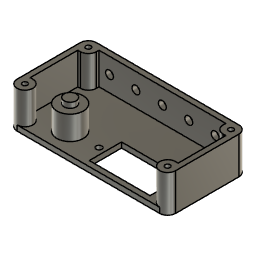
TRGRIP01_Base_Top_60x30x14 (Autodesk Fusion 360 design; units mm, degrees)
Autodesk Fusion 360 part; units mm, degrees
sketch "스케치1" plane through (0, 0, 0) normal (0, 0, 1) x (1, 0, 0)
  line L0 (0, 0) -> (60, 0)
  line L1 (60, 0) -> (60, 30)
  line L2 (60, 30) -> (0, 30)
  line L3 (0, 30) -> (0, 0)
  dimension "d1" = 60
  dimension "d2" = 30
  constraint horizontal L0
  constraint vertical L1
  constraint horizontal L2
  constraint vertical L3
  constraint coincident L0.start L3.end
  measures "d1" distance of L0.start L0.end
  measures "d2" distance of L0.start L2.end
extrude "돌출1" add sketch "스케치1" along normal blind 2
sketch "스케치2" plane through (0, 0, 2) normal (0, 0, 1) x (-1, 0, 0)
  circle A0 centre (-53.75, -8.1) radius 1.1
  circle A1 centre (-25.95, -8.1) radius 1.1
  circle A2 centre (-15, -8.1) radius 5
  line L0 (0, 0) -> (-60, 0)
  line L1 (-51.35, -2) -> (-51.35, -14.2)
  line L2 (-51.35, -14.2) -> (-28.35, -14.2)
  line L3 (-28.35, -14.2) -> (-28.35, -2)
  line L4 (-51.35, -2) -> (-28.35, -2)
  dimension "d5" = 2.2
  dimension "d6" = 27.8
  dimension "d8" = 8.1
  dimension "d9" = 10
  dimension "d11" = 15
  dimension "d28" = 25.95
  dimension "d91" = 23
  dimension "d93" = 2.4
  dimension "d94" = 2
  dimension "d95" = 12.2
  constraint equal A0 A1
  constraint horizontal A0.centre A1.centre
  constraint vertical L1
  constraint horizontal L2
  constraint vertical L3
  constraint horizontal A1.centre A2.centre
  constraint perpendicular L3 L4
  measures "d5" diameter of A0
  measures "d6" distance of A0.centre A1.centre
  measures "d8" vertical distance of L0.start A0.centre
  measures "d9" diameter of A2
  measures "d11" horizontal distance of L0.start A2.centre
  measures "d28" horizontal distance of L0.start A1.centre
  measures "d91" distance of L1 L3
  measures "d93" horizontal distance of A1.centre L3.end
  measures "d94" vertical distance of L0.start L1.start
  measures "d95" distance of L2.end L3.end
extrude "돌출2" cut sketch "스케치2" against normal blind 2 contours A0 | A1 | L1 L2 L3 L4
extrude "돌출3" add sketch "스케치2" along normal blind 9 contours A2
sketch "스케치4" plane through (0, 0, 11) normal (0, 0, 1) x (-1, 0, 0)
  circle A0 centre (-15, -8.1) radius 2.3
  circle A1 centre (-15, -8.1) radius 5
  dimension "d34" = 4.6
  constraint concentric A0 A1
  measures "d34" diameter of A0
extrude "돌출5" add sketch "스케치4" along normal blind 2 contours A0
sketch "스케치5" plane through (0, 0, 2) normal (0, 0, 1) x (-1, 0, 0)
  line L0 (0, -30) -> (0, 0)
  line L1 (0, 0) -> (0, -30)
  line L2 (-60, -30) -> (0, -30)
  line L3 (-60, -30) -> (-60, 0)
  line L4 (0, 0) -> (-60, 0)
  line L5 (-60, 0) -> (-54, 0)
  line L6 (-54, -28) -> (-6, -28)
  line L7 (-2, -24) -> (-2, -6)
  line L8 (-6, 0) -> (0, 0)
  line L9 (-58, -24) -> (-58, -6)
  line L10 (-2, -24) -> (-6, -24)
  line L11 (-6, -24) -> (-6, -28)
  line L12 (-54, -28) -> (-54, -24)
  line L13 (-54, -24) -> (-58, -24)
  line L14 (-2, -6) -> (-6, -6)
  line L15 (0, 0) -> (-60, 0)
  line L16 (-6, -6) -> (-6, 0)
  line L17 (-58, -6) -> (-54, -6)
  line L18 (-54, -6) -> (-54, 0)
  point P0 (0, -30)
  point P1 (-60, -30)
  point P2 (-60, 0)
  dimension "d38" = 2
  dimension "d39" = 2
  dimension "d42" = 2
  dimension "d43" = 6
  dimension "d44" = 6
  dimension "d45" = 6
  dimension "d46" = 6
  dimension "d47" = 6
  constraint coincident L0.end L1.start
  constraint coincident P0 L0.start
  constraint coincident P1 L2.start
  constraint coincident P2 L3.end
  constraint coincident L4 L5.end
  constraint perpendicular L0 L5
  constraint perpendicular L0 L6
  constraint perpendicular L6 L7
  constraint perpendicular L1 L8
  constraint perpendicular L5 L9
  constraint perpendicular L7 L10
  constraint perpendicular L10 L11
  constraint perpendicular L6 L12
  constraint perpendicular L9 L13
  constraint perpendicular L7 L14
  constraint coincident L15 L8.start
  constraint perpendicular L15 L16
  constraint perpendicular L9 L17
  constraint perpendicular L4 L18
  constraint equal L10 L14
  constraint equal L11 L12
  constraint equal L13 L17
  measures "d38" distance of L2 L6
  measures "d39" distance of L3 L9
  measures "d42" distance of L1 L7
  measures "d43" distance of L0.end L8.start
  measures "d44" vertical distance of L0.end L14.end
  measures "d45" distance of P2 L5.end
  measures "d46" distance of L17.end L5.end
  measures "d47" vertical distance of P0 L10.end
extrude "돌출6" add sketch "스케치5" along normal blind 12 contours L0 L1 L2 L3 L4 L5 L6 L7 L8 L9 L10 L11 L12 L13 L14 L15 L16 L17 L18
sketch "스케치6" plane through (0, 0, 14) normal (0, 0, 1) x (-1, 0, 0)
  circle A0 centre (-3, -27) radius 0.95
  circle A1 centre (-3, -3) radius 0.95
  circle A2 centre (-57, -27) radius 0.95
  circle A3 centre (-57, -3) radius 0.95
  dimension "d48" = 1.9
  dimension "d49" = 3
  dimension "d51" = 3
  dimension "d52" = 24
  dimension "d53" = 54
  constraint equal A2 A3
  constraint equal A0 A2
  constraint equal A0 A1
  constraint vertical A0.centre A1.centre
  constraint horizontal A0.centre A2.centre
  constraint vertical A2.centre A3.centre
  constraint horizontal A1.centre A3.centre
  measures "d48" diameter of A0
  measures "d49" horizontal distance of origin A1.centre
  measures "d51" vertical distance of origin A1.centre
  measures "d52" distance of A0.centre A1.centre
  measures "d53" distance of A0.centre A2.centre
extrude "돌출7" cut sketch "스케치6" against normal blind 5
fillet "필렛1" radius 3 8 edges at (60, 0, 7) (0, 0, 7) (60, 30, 7) (0, 30, 7) (54, 24, 8) (6, 24, 8) (54, 6, 8) (6, 6, 8)
fillet "필렛1" radius 3 2 edges at (54, 0, 8) (6, 0, 8)
sketch "스케치9" plane through (0, 30, 0) normal (0, 1, 0) x (-1, 0, 0)
  circle A0 centre (-50, 8) radius 1.5
  circle A1 centre (-30, 8) radius 1.5
  circle A2 centre (-10, 8) radius 1.5
  circle A3 centre (-40, 8) radius 1.5
  circle A4 centre (-20, 8) radius 1.5
  dimension "d74" = 3
  dimension "d75" = 8
  dimension "d80" = 10
  dimension "d81" = 10
  dimension "d82" = 10
  dimension "d83" = 10
  dimension "d84" = 10
  constraint horizontal A0.centre A1.centre
  constraint equal A0 A1
  constraint equal A1 A2
  constraint horizontal A1.centre A2.centre
  constraint equal A1 A3
  constraint equal A1 A4
  constraint horizontal A1.centre A3.centre
  constraint horizontal A3.centre A4.centre
  measures "d74" diameter of A0
  measures "d75" vertical distance of origin A1.centre
  measures "d80" horizontal distance of origin A2.centre
  measures "d81" distance of A2.centre A4.centre
  measures "d82" distance of A1.centre A4.centre
  measures "d83" distance of A1.centre A3.centre
  measures "d84" distance of A0.centre A3.centre
extrude "돌출10" cut sketch "스케치9" against normal blind 2
